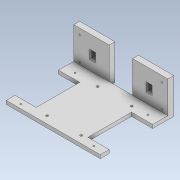
# Autodesk Inventor part: electrical_system_fix_board
Saved by Autodesk Inventor 2020 (Build 240168000, 168)
## iProperties
Created: 2021-01-08
Part Number: electrical_system_fix_board
Material: Generic
Document SubType Name: Modeling
Designer: DELL
Density: 1 g/cm^3
Appearance: Default
Author: DELL
Autodesk Inventor part; units mm, degrees
ref_plane "YZ Plane" through (0, 0, 0) normal (1, 0, 0) x (0, 1, 0)
ref_plane "XZ Plane" through (0, 0, 0) normal (0, 1, 0) x (-1, 0, 0)
ref_plane "XY Plane" through (0, 0, 0) normal (0, 0, 1) x (1, 0, 0)
sketch "Sketch1" plane through (0, 0, 0) normal (0, 0, 1) x (1, 0, 0)
  line L0 (80, 30) -> (-80, 30)
  line L1 (-80, 30) -> (-80, -30)
  line L2 (-80, -30) -> (80, -30)
  line L3 (80, -30) -> (80, 30)
  line L4 (80, 30) -> (-80, -30) construction
  line L5 (-80, 30) -> (80, -30) construction
  line L6 (-20, -30) -> (-80, -30)
  line L7 (-80, -30) -> (-80, 30)
  line L8 (-80, 30) -> (-20, 30)
  line L9 (-20, 30) -> (-20, -30)
  line L10 (-20, -30) -> (-80, 30) construction
  line L11 (-80, -30) -> (-20, 30) construction
  line L12 (20, -30) -> (80, -30)
  line L13 (80, -30) -> (80, 30)
  line L14 (80, 30) -> (20, 30)
  line L15 (20, 30) -> (20, -30)
  line L16 (20, -30) -> (80, 30) construction
  line L17 (80, -30) -> (20, 30) construction
  line L18 (0, 30) -> (0, -30) construction
  point P0 (0, 0)
  point P1 (-50, 0)
  point P2 (50, 0)
  point P3 (20, 30)
  point P4 (20, -30)
  point P5 (-20, -30)
  point P6 (-20, 30)
  dimension "d0" = 160
  dimension "d1" = 60
  dimension "d2" = 40
  constraints: 38 end point, 8 midpoint, 6 parallel, 3 horizontal, 3 perpendicular, 2 collinear, 1 other
  measures "d0" distance between parallel lines of L3 L1
  measures "d1" distance between parallel lines of L2 L0
  measures "d2" distance between parallel lines of L15 L9
extrude "Extrusion1" add sketch "Sketch1" along normal blind 10 contours L3 L2 L15 L0 | L9 L2 L1 L0
sketch "Sketch2" plane through (0, 0, 10) normal (0, 0, 1) x (1, 0, 0)
  line L0 (-80, -30) -> (-20, -30) projected
  line L1 (80, -24) -> (-80, -24)
  line L2 (-80, -24) -> (-80, -30)
  line L3 (-80, -30) -> (80, -30)
  line L4 (80, -30) -> (80, -24)
  line L5 (80, -24) -> (-80, -30) construction
  line L6 (-80, -24) -> (80, -30) construction
  line L7 (80, -30) -> (80, 30) projected
  point P0 (0, 0)
  point P1 (0, -27)
  dimension "d5" = 6
  constraints: 12 end point, 2 midpoint, 2 parallel, 1 collinear, 1 horizontal, 1 perpendicular
  measures "d5" distance between parallel lines of L3 L1
extrude "Extrusion2" add sketch "Sketch2" along normal blind 115
sketch "Sketch3" plane through (0, 0, 0) normal (0, 0, -1) x (-1, 0, 0)
  line L0 (53, 7.5) -> (43, 7.5)
  line L1 (43, 7.5) -> (43, -7.5)
  line L2 (43, -7.5) -> (53, -7.5)
  line L3 (53, -7.5) -> (53, 7.5)
  line L4 (53, 7.5) -> (43, -7.5) construction
  line L5 (43, 7.5) -> (53, -7.5) construction
  line L6 (-43, 7.5) -> (-53, 7.5)
  line L7 (-53, 7.5) -> (-53, -7.5)
  line L8 (-53, -7.5) -> (-43, -7.5)
  line L9 (-43, -7.5) -> (-43, 7.5)
  line L10 (-43, 7.5) -> (-53, -7.5) construction
  line L11 (-53, 7.5) -> (-43, -7.5) construction
  line L12 (80, -30) -> (-80, -30) construction
  line L13 (0, -30) -> (0, 0) construction
  point P0 (48, 0)
  point P1 (-48, 0)
  point P2 (48, 0)
  dimension "d8" = 10
  dimension "d9" = 15
  dimension "d10" = 48
  constraints: 26 end point, 6 midpoint, 4 parallel, 2 equal length, 2 horizontal, 2 perpendicular, 1 horizontal alignment, 1 vertical, 2 other
  measures "d8" distance of L1.end L2.end
  measures "d9" distance of L2.end L0.start
  measures "d10" distance from line of L13 point (48, 0)
extrude "Extrusion3" cut sketch "Sketch3" against normal through all
sketch "Sketch4" plane through (0, 0, 0) normal (0, 0, -1) x (-1, 0, 0)
  line L0 (-70, -20) -> (70, -20) construction
  line L1 (70, -20) -> (70, 20) construction
  line L2 (70, 20) -> (-70, 20) construction
  line L3 (-70, 20) -> (-70, -20) construction
  line L4 (-70, -20) -> (70, 20) construction
  line L5 (70, -20) -> (-70, 20) construction
  circle A0 centre (70, 20) radius 1.25
  circle A1 centre (-70, 20) radius 1.25
  circle A2 centre (-70, -20) radius 1.25
  circle A3 centre (70, -20) radius 1.25
  point P0 (0, 0)
  dimension "d13" = 140
  dimension "d14" = 40
  dimension "d16" = 2.5
  constraints: 12 end point, 4 centre point, 4 coincident, 3 equal radius, 2 midpoint, 2 parallel, 1 horizontal, 1 perpendicular
  measures "d13" distance of L1.end L2.end
  measures "d14" distance of L0.end L1.end
  measures "d16" diameter of A0
extrude "Extrusion4" cut sketch "Sketch4" against normal through all
sketch "Sketch5" plane through (-20, -24, 10) normal (0, 1, 0) x (1, 0, 0)
  line L0 (59.5, -13) -> (-19.5, -13) construction
  line L1 (-19.5, -13) -> (-19.5, -113) construction
  line L2 (-19.5, -113) -> (59.5, -113) construction
  line L3 (59.5, -113) -> (59.5, -13) construction
  line L4 (59.5, -13) -> (-19.5, -113) construction
  line L5 (-19.5, -13) -> (59.5, -113) construction
  line L6 (100, -115) -> (-60, -115) construction
  line L7 (55.5, -17) -> (-2.5, -17) construction
  line L8 (-2.5, -17) -> (-2.5, -103) construction
  line L9 (-2.5, -103) -> (55.5, -103) construction
  line L10 (55.5, -103) -> (55.5, -17) construction
  line L11 (55.5, -17) -> (-2.5, -103) construction
  line L12 (-2.5, -17) -> (55.5, -103) construction
  circle A0 centre (-2.5, -17) radius 1.75
  circle A1 centre (55.5, -17) radius 1.75
  circle A2 centre (-2.5, -103) radius 1.75
  circle A3 centre (55.5, -103) radius 1.75
  line L13 (-60, -26) -> (-24, -26)
  line L14 (-24, -26) -> (-24, -100)
  line L15 (-24, -100) -> (-60, -100)
  line L16 (-60, -100) -> (-60, -26)
  line L17 (-60, -26) -> (-24, -100) construction
  line L18 (-24, -26) -> (-60, -100) construction
  line L19 (100, -26) -> (64, -26)
  line L20 (64, -26) -> (64, -100)
  line L21 (64, -100) -> (100, -100)
  line L22 (100, -100) -> (100, -26)
  line L23 (100, -26) -> (64, -100) construction
  line L24 (64, -26) -> (100, -100) construction
  line L25 (20, 10) -> (20, -115) construction
  line L26 (-60, 0) -> (-60, -115) construction
  circle A4 centre (-42, -16) radius 1.25
  circle A5 centre (-42, -108) radius 1.25
  circle A6 centre (82, -16) radius 1.25
  circle A7 centre (82, -108) radius 1.25
  line L27 (-60, 10) -> (-60, -115) construction
  line L28 (-60, -63) -> (100, -63) construction
  line L29 (0, 0) -> (-60, 0) projected
  point P0 (20, -63)
  point P1 (20, -63)
  point P2 (26.5, -60)
  point P3 (20, -63)
  point P4 (26.5, -60)
  point P5 (-42, -63)
  point P6 (82, -63)
  point P7 (-42, -63)
  point P8 (82, -63)
  point P9 (-42, -63)
  point P10 (82, -63)
  dimension "d20" = 79
  dimension "d21" = 100
  dimension "d22" = 58
  dimension "d23" = 86
  dimension "d26" = 4
  dimension "d27" = 4
  dimension "d28" = 3.5
  dimension "d31" = 36
  dimension "d32" = 74
  dimension "d36" = 2.5
  dimension "d39" = 13
  dimension "d42" = 4.5
  dimension "d43" = 45
  dimension "d44" = 47
  constraints: 52 end point, 18 midpoint, 8 centre point, 8 parallel, 6 equal radius, 4 coincident, 4 horizontal, 4 horizontal alignment, 4 perpendicular, 4 vertical alignment, 2 equal length, 2 point on line, 1 collinear, 1 other
  measures "d20" distance between parallel lines of L3 L1
  measures "d21" distance between parallel lines of L2 L0
  measures "d22" distance of L7.start L7.end
  measures "d23" distance of L9.end L7.start
  measures "d26" distance between parallel lines of L3 L10
  measures "d27" distance between parallel lines of L0 L7
  measures "d28" diameter of A0
  measures "d31" distance of L13.start L13.end
  measures "d32" distance of L15.end L13.start
  measures "d36" diameter of A4
  measures "d39" distance between parallel lines of L29 L0
  measures "d42" distance between parallel lines of L14 L1
  measures "d43" distance from line of L28 A5.centre
  measures "d44" distance from line of L28 A4.centre
extrude "Extrusion5" cut sketch "Sketch5" against normal through all contours A0 | A1 | A2 | A3
extrude "Extrusion6" cut sketch "Sketch5" against normal through all contours L13 L14 L15 L16 | L22 L21 L20 L19
extrude "Extrusion7" cut sketch "Sketch5" against normal through all contours A4 | A5 | A6 | A7
body "Solid1"
